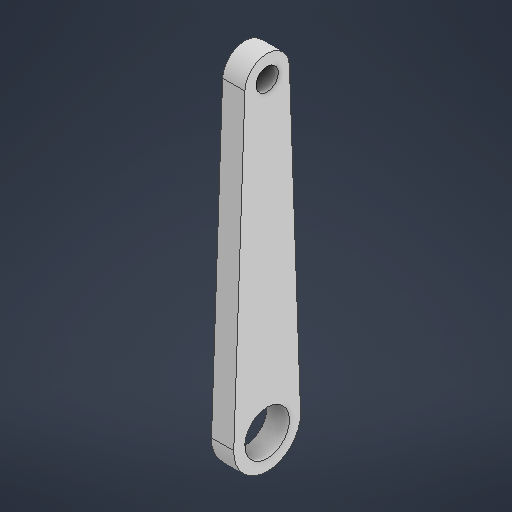
# Autodesk Inventor part: crank
Saved by Autodesk Inventor 2026.2 (Build 302298010, 298A)
## iProperties
Created: 2026-07-07
Part Number: crank
Material: Generic
Document SubType Name: Modeling
Designer: tasle
Density: 1 g/cm^3
Appearance: Default
Author: tasle
Autodesk Inventor part; units mm, degrees
ref_plane "YZ Plane" through (0, 0, 0) normal (1, 0, 0) x (0, 1, 0)
ref_plane "XZ Plane" through (0, 0, 0) normal (0, 1, 0) x (-1, 0, 0)
ref_plane "XY Plane" through (0, 0, 0) normal (0, 0, 1) x (1, 0, 0)
sketch "Sketch1" plane through (0, 0, 0) normal (1, 0, 0) x (0, 1, 0)
  circle A0 centre (0, 0) radius 4
  circle A1 centre (0, 0) radius 6
  circle A2 centre (55, 0) radius 2
  circle A3 centre (55, 0) radius 4
  line L0 (55, 0) -> (0, 0)
  line L1 (55.1455, 3.9974) -> (0.2182, 5.996)
  line L2 (55.1455, -3.9974) -> (0.2182, -5.996)
  dimension "d0" = 8
  dimension "d1" = 12
  dimension "d2" = 4
  dimension "d3" = 8
  dimension "d4" = 55
  constraints: 6 end point, 4 centre point, 4 point on circle, 4 tangent, 3 coincident, 1 horizontal
  measures "d0" diameter of A0
  measures "d1" diameter of A1
  measures "d2" diameter of A2
  measures "d3" diameter of A3
  measures "d4" distance of L0.start L0.end
extrude "Extrusion1" add sketch "Sketch1" along normal blind 4
body "Solid1"
